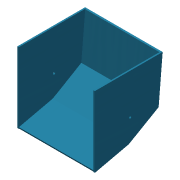
# Autodesk Inventor part: Bucket
Saved by Autodesk Inventor 2013 (Build 170138000, 138)
## iProperties
Created: 2014-01-16
Part Number: Bucket
Material: Generic
Document SubType Name: Modeling
Designer: rihoobler
Density: 1 g/cm^3
Author: rihoobler
Autodesk Inventor part; units mm, degrees
ref_plane "YZ Plane" through (0, 0, 0) normal (1, 0, 0) x (0, 1, 0)
ref_plane "XZ Plane" through (0, 0, 0) normal (0, 1, 0) x (-1, 0, 0)
ref_plane "XY Plane" through (0, 0, 0) normal (0, 0, 1) x (1, 0, 0)
sketch "Sketch1" plane through (0, 0, 0) normal (1, 0, 0) x (0, 1, 0)
  line L0 (-63.8691, 100.7559) -> (-60.6941, 100.7559)
  line L1 (-12.0126, 2.1649) -> (-29.1539, 76.4119)
  line L2 (-12.0126, 2.1649) -> (64.1874, 2.1649) construction
  line L3 (-12.0126, 2.1649) -> (26.0874, -63.8262)
  line L4 (-12.0126, 2.1649) -> (64.1874, 2.1649) construction
  line L5 (26.0874, -63.8262) -> (127.3008, -72.6812)
  line L6 (-29.1539, 76.4119) -> (-26.0603, 77.1261)
  line L7 (-26.0603, 77.1261) -> (-8.7541, 2.1649)
  line L8 (127.3008, -72.6812) -> (126.5865, -69.5876)
  line L9 (126.5865, -69.5876) -> (28.235, -60.983)
  line L10 (1.2031, -15.1211) -> (28.235, -60.983)
  line L11 (1.2031, -15.1211) -> (-8.7541, 2.1649)
  dimension "d4" = 3.175
  dimension "d6" = 76.2
  dimension "d7" = 103
  dimension "d8" = 76.2
  dimension "d9" = 60
  dimension "d10" = 101.6
  dimension "d11" = 125
  dimension "d12" = 3.175
  dimension "d13" = 3.175
  constraints: 24 end point, 2 equal length, 2 horizontal, 2 parallel, 2 perpendicular, 1 point on line
  measures "d4" distance of L0.start L0.end
  measures "d6" distance of L1.start L1.end
  measures "d7" angle of L2 L1
  measures "d8" distance of L1.start L3.end
  measures "d9" angle of L3 L4
  measures "d10" distance of L3.end L5.end
  measures "d11" angle of L5 L3
  measures "d12" distance of L1.end L6.end
  measures "d13" distance of L5.end L8.end
extrude "Extrusion1" add sketch "Sketch1" along normal mid plane 165.1
sketch "Sketch2" plane through (82.55, 0, 0) normal (1, 0, 0) x (0, 0, -1)
  line L0 (63.8262, 26.0874) -> (72.6812, 127.3008) projected
  line L1 (69.5876, 126.5865) -> (60.983, 28.235) projected
  line L2 (72.6812, 127.3008) -> (-77.2337, 127.3008)
  line L3 (-77.2337, 127.3008) -> (-77.2337, -29.1539)
  line L4 (-77.2337, -29.1539) -> (-76.4119, -29.1539)
  line L5 (72.6812, 127.3008) -> (63.8262, 26.0874)
  line L6 (-76.4119, -29.1539) -> (-2.1649, -12.0126) projected
  line L7 (-2.1649, -12.0126) -> (63.8262, 26.0874) projected
  line L8 (-76.4119, -29.1539) -> (-2.1649, -12.0126)
  line L9 (-2.1649, -12.0126) -> (63.8262, 26.0874)
  point P0 (0, 0)
  constraints: 12 end point, 2 collinear, 1 parallel, 1 perpendicular
extrude "Extrusion2" add sketch "Sketch2" along normal blind 3.175
sketch "Sketch3" plane through (-82.55, 0, 0) normal (-1, 0, 0) x (0, 0, 1)
  line L0 (-69.5876, 126.5865) -> (-72.6812, 127.3008) projected
  line L1 (-72.6812, 127.3008) -> (-63.8262, 26.0874) projected
  line L2 (-63.8262, 26.0874) -> (2.1649, -12.0126) projected
  line L3 (77.2337, -29.1539) -> (-72.6812, -29.1539)
  line L4 (-72.6812, -29.1539) -> (-72.6812, 127.3008)
  line L5 (-72.6812, 127.3008) -> (77.2337, 127.3008)
  line L6 (77.2337, 127.3008) -> (77.2337, -29.1539)
  line L7 (-72.6812, 127.3008) -> (-63.8262, 26.0874)
  line L8 (-63.8262, 26.0874) -> (2.1649, -12.0126)
  line L9 (2.1649, -12.0126) -> (76.4119, -29.1539)
  line L10 (76.4119, -29.1539) -> (77.2337, -29.1539)
  point P0 (0, 0)
  constraints: 16 end point, 3 parallel, 2 collinear, 1 horizontal, 1 perpendicular, 1 point on line
extrude "Extrusion3" add sketch "Sketch3" along normal blind 3.175 contours L5 L6 L3 L9 L2 L1
sketch "Sketch4" plane through (-82.55, 0, 0) normal (1, 0, 0) x (0, 0, -1)
  circle A0 centre (1.1115, 38.0788) radius 2.413
  point P0 (0, 0)
  dimension "d21" = 4.826
  constraints: 1 centre point, 1 coincident
  measures "d21" diameter of A0
extrude "Extrusion4" cut sketch "Sketch4" along normal through all both and the other way through all
body "Solid1"
